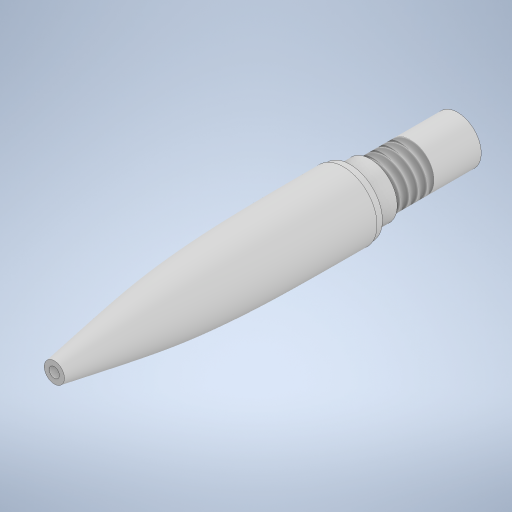
# Autodesk Inventor part: 筆頭
Saved by Autodesk Inventor 2024.2 (Build 282272000, 272)
## iProperties
Created: 2024-04-18
Part Number: 筆頭
Material: 一般
Document SubType Name: Modeling
Designer: User
Density: 1 g/cm^3
Appearance: 預設
Author: User
Autodesk Inventor part; units mm, degrees
ref_plane "YZ Plane" through (0, 0, 0) normal (1, 0, 0) x (0, 1, 0)
ref_plane "XZ Plane" through (0, 0, 0) normal (0, 1, 0) x (-1, 0, 0)
ref_plane "XY Plane" through (0, 0, 0) normal (0, 0, 1) x (1, 0, 0)
sketch "草圖1" plane through (0, 0, 0) normal (0, 1, 0) x (-1, 0, 0)
  line L0 (0, 0) -> (0, -56)
  line L1 (0, 0) -> (1.5, 0)
  line L2 (0, -60) -> (3, -60)
  line L3 (4, -44) -> (4, -47)
  line L4 (4, -60) -> (4, -60)
  line L5 (1.5, 0) -> (2.8279, -7.7525) construction
  line L6 (2.8279, -7.7525) -> (4, -14.5952) construction
  line L7 (4, -14.5952) -> (4.4961, -20.3364) construction
  line L8 (4.8, -43) -> (4.8, -44)
  line L9 (4.8, -43) -> (4.9998, -43) construction
  line L10 (4.9998, -43) -> (5, -43) construction
  line L11 (4.8, -43) -> (4.9998, -43)
  line L12 (4.8, -44) -> (4, -44)
  spline S0 degree 4 poles (1.5, 0) (2.8279, -7.7525) (4, -14.5952) (4.4961, -20.3364) (4.855, -25.9559) (4.9951, -32.7037) (4.9998, -43) knots 1 1 1 1 1 2 3 3.976846 3.976846 3.976846 3.976846 3.976846
  line L13 (4.4961, -20.3364) -> (4.855, -25.9559) construction
  line L14 (4.855, -25.9559) -> (4.9951, -32.7037) construction
  line L15 (4.9951, -32.7037) -> (4.9998, -43) construction
  line L16 (0, -60) -> (0, -56)
  line L17 (0, -56) -> (3.5, -56)
  line L18 (0, -56) -> (0, -60)
  line L19 (4, -44) -> (4, -47)
  line L20 (4, -47) -> (3.5, -47)
  line L21 (3.5, -47) -> (3.5, -56)
  line L22 (3.5, -47) -> (0, -47)
  line L23 (3.5, -56) -> (3, -56)
  line L24 (3, -56) -> (3, -60)
  line L25 (3.5, -56) -> (3.5, -60)
  line L26 (3.5, -60) -> (3, -60)
  dimension "d0" = 60
  dimension "d1" = 1.5
  dimension "d5" = 16
  dimension "d6" = 4
  dimension "d12" = 0.8
  dimension "d13" = 0.1998
  dimension "d14" = 4
  dimension "d15" = 3
  dimension "d16" = 0.5
  dimension "d17" = 0.5
  constraints: 42 end point, 10 perpendicular, 5 horizontal, 2 point on line, 2 vertical, 1 parallel, 3 other
  measures "d0" distance of L0.start L2.start
  measures "d1" distance of L0.start L1.end
  measures "d5" distance of L3.start L4.start
  measures "d6" distance of L2.start L4.start
  measures "d12" distance of L8.end L3.start
  measures "d13" distance of L8.start L9.end
  measures "d14" distance of L2.start L0.end
  measures "d15" distance of L3.end L3.start
  measures "d16" distance of L3.end L20.end
  measures "d17" distance of L17.end L23.end
revolve "迴轉1" add sketch "草圖1" angle 360 about axis through (0, 0, 0) along (0, 0, -1)
thread "螺紋1" size "G16.662x1.337" designation "G 3/8" class "A" standard "ISO Pipe Threads" length 6
shell "薄殼1" thickness 1 removed faces 2 at (-3.2994, -0.2792, -60) at (0.7485, -0.6631, -60)
sketch "草圖2" plane through (0, 0, 0) normal (0, 0, 1) x (1, 0, 0)
  point P0 (0, 0)
  point P1 (0, 0)
  constraints: 1 coincident
hole "孔1" at (0, 0, 0) direction (0, 0, -1) diameter 1.5 depth 14.5 tip angle 118
